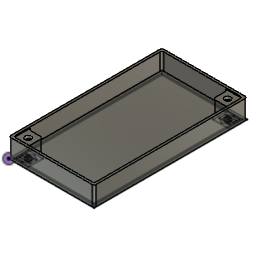
assemblage v25 (Autodesk Fusion 360 archive; units mm, degrees)
design "basBoite"
Autodesk Fusion 360 part; units mm, degrees
sketch "Sketch1" plane through (0, 0, 0) normal (0, 0, 1) x (1, 0, 0)
  line L0 (0, 0) -> (44, 0)
  line L1 (44, 0) -> (44, 79)
  line L2 (44, 79) -> (0, 79)
  line L3 (0, 79) -> (0, 0)
  line L4 (1.2, 1.2) -> (42.8, 1.2)
  line L5 (42.8, 1.2) -> (42.8, 77.8)
  line L6 (42.8, 77.8) -> (1.2, 77.8)
  line L7 (1.2, 77.8) -> (1.2, 1.2)
  line L8 (42, 2) -> (42, 77)
  line L9 (42, 77) -> (2, 77)
  line L10 (2, 77) -> (2, 2)
  line L11 (2, 2) -> (42, 2)
  line L12 (1.2, 1.2) -> (8.8, 1.2)
  line L13 (8.8, 1.2) -> (8.8, 8.8)
  line L14 (8.8, 8.8) -> (1.2, 8.8)
  line L15 (1.2, 8.8) -> (1.2, 1.2)
  line L16 (2, 2) -> (5, 2)
  line L17 (5, 2) -> (5, 5)
  line L18 (5, 5) -> (2, 5)
  line L19 (2, 5) -> (2, 2)
  circle A0 centre (5, 5) radius 1.6
  line L20 (7.75, 6.5877) -> (5, 8.1754)
  line L21 (5, 8.1754) -> (2.25, 6.5877)
  line L22 (2.25, 6.5877) -> (2.25, 3.4123)
  line L23 (2.25, 3.4123) -> (5, 1.8246)
  line L24 (5, 1.8246) -> (7.75, 3.4123)
  line L25 (7.75, 3.4123) -> (7.75, 6.5877)
  line L26 (2.25, 6.6) -> (7.75, 6.6)
  line L27 (2.25, 3.4) -> (7.75, 3.4)
  line L28 (6.6, 6.6) -> (6.6, 3.4)
  line L29 (3.4, 6.6) -> (3.4, 3.4)
  line L30 (42.8, 77.8) -> (35.2, 77.8)
  line L31 (35.2, 77.8) -> (35.2, 70.2)
  line L32 (35.2, 70.2) -> (42.8, 70.2)
  line L33 (42.8, 70.2) -> (42.8, 77.8)
  line L34 (42, 77) -> (39, 77)
  line L35 (39, 77) -> (39, 74)
  line L36 (39, 74) -> (42, 74)
  line L37 (42, 74) -> (42, 77)
  circle A1 centre (39, 74) radius 1.6
  line L38 (36.25, 72.4123) -> (39, 70.8246)
  line L39 (39, 70.8246) -> (41.75, 72.4123)
  line L40 (41.75, 72.4123) -> (41.75, 75.5877)
  line L41 (41.75, 75.5877) -> (39, 77.1754)
  line L42 (39, 77.1754) -> (36.25, 75.5877)
  line L43 (36.25, 75.5877) -> (36.25, 72.4123)
  line L44 (36.25, 75.6) -> (41.75, 75.6)
  line L45 (36.25, 72.4) -> (41.75, 72.4)
  line L46 (37.4, 75.6) -> (37.4, 72.4)
  line L47 (40.6, 75.6) -> (40.6, 72.4)
  point P0 (5, 5)
  point P1 (39, 74)
  dimension "d1" = 44
  dimension "d2" = 79
  dimension "d3" = -1.2
  dimension "d4" = -2
  dimension "d35" = 7.6
  dimension "d36" = 7.6
  dimension "d37" = 3
  dimension "d38" = 3
  dimension "d39" = 3.2
  dimension "d40" = 2.75
  dimension "d41" = 7.6
  dimension "d42" = 7.6
  dimension "d43" = 3
  dimension "d44" = 3
  dimension "d45" = 3.2
  dimension "d46" = 2.75
  constraint horizontal L0
  constraint vertical L1
  constraint horizontal L2
  constraint vertical L3
  constraint coincident L0.start L3.end
  constraint horizontal L12
  constraint vertical L13
  constraint horizontal L14
  constraint vertical L15
  constraint horizontal L16
  constraint vertical L17
  constraint horizontal L18
  constraint vertical L19
  constraint coincident P0 L17.end
  constraint coincident L22 L26.start
  constraint coincident L25 L26.end
  constraint perpendicular L25 L26
  constraint coincident L22 L27.start
  constraint coincident L25 L27.end
  constraint perpendicular L25 L27
  constraint tangent A0 L26
  constraint tangent A0 L27
  constraint coincident L26 L28.start
  constraint coincident L27 L28.end
  constraint perpendicular L27 L28
  constraint coincident L26 L29.start
  constraint coincident L27 L29.end
  constraint perpendicular L27 L29
  constraint tangent A0 L29
  constraint tangent A0 L28
  constraint horizontal L30
  constraint vertical L31
  constraint horizontal L32
  constraint vertical L33
  constraint horizontal L34
  constraint vertical L35
  constraint horizontal L36
  constraint vertical L37
  constraint coincident P1 L35.end
  constraint coincident L43 L44.start
  constraint coincident L40 L44.end
  constraint perpendicular L40 L44
  constraint coincident L43 L45.start
  constraint coincident L40 L45.end
  constraint perpendicular L40 L45
  constraint tangent A1 L44
  constraint tangent A1 L45
  constraint coincident L44 L46.start
  constraint coincident L45 L46.end
  constraint perpendicular L45 L46
  constraint coincident L44 L47.start
  constraint coincident L45 L47.end
  constraint perpendicular L45 L47
  constraint tangent A1 L46
  constraint tangent A1 L47
  constraint vertical L25
  constraint vertical L43
  measures "d1" distance of L0.start L0.end
  measures "d2" distance of L0.start L2.end
  measures "d35" distance of L4.start L12.end
  measures "d36" distance of L4.start L14.end
  measures "d37" distance of L10.end L16.end
  measures "d38" distance of L10.end L18.end
  measures "d39" diameter of A0
  measures "d40" distance of P0 L25
  measures "d41" distance of L5.end L30.end
  measures "d42" distance of L5.end L32.end
  measures "d43" distance of L8.end L34.end
  measures "d44" distance of L8.end L36.end
  measures "d45" diameter of A1
  measures "d46" distance of P1 L43
extrude "Extrude21" add sketch "Sketch1" along normal blind 1.2 contours L4 L5 L8 L11 L13 L32 | L6 L7 L9 L10 L14 L31 | L8 L9 L10 L11 L13 L14 L31 L32
extrude "Extrude22" add sketch "Sketch1" along normal blind 10
extrude "Extrude23" add sketch "Sketch1" along normal blind 9 contours L5 L6 L8 L9 L30 L31 L32 L33 L34 L37 L41 L42 | L8 L9 L31 L32 L36 L38 L39 L40 L42 L43 | L8 L9 L34 L36 L37 L40 L41 | L9 L35 L42 L44 | L36 L39 L40 L45 L47 | L36 L40 L41 L44 L47 | L9 L34 L35 L41 L44 | L38 L42 L43 L44 L45 L46 | A1 L45 L47 | A1 L44 L47 | A1 L44 L46 | A1 L45 L46 | L38 L39 L45
extrude "Extrude24" add sketch "Sketch1" along normal blind 9 contours L9 L34 L41 L42
extrude "Extrude25" cut sketch "Sketch1" along normal blind 7.8 contours A1 L45 L47 | A1 L44 L47 | A1 L44 L46 | A1 L45 L46
extrude "Extrude26" cut sketch "Sketch1" along normal blind 7.5 contours L36 L39 L40 L45 L47 | L36 L40 L41 L44 L47 | L38 L42 L43 L44 L45 L46
extrude "Extrude27" cut sketch "Sketch1" along normal blind 7.2 contours L9 L34 L41 L42 | L9 L35 L42 L44 | L9 L34 L35 L41 L44 | L38 L39 L45
extrude "Extrude28" add sketch "Sketch1" along normal blind 9 contours L4 L7 L10 L11 L12 L13 L14 L15 L16 L19 L23 L24 | L10 L11 L13 L14 L18 L20 L21 L22 L24 L25 | L11 L16 L23 L24 | L11 L17 L24 L27 | L10 L11 L16 L18 L19 L22 L23 | L11 L16 L17 L23 L27 | L20 L24 L25 L26 L27 L28 | L18 L21 L22 L26 L29 | L18 L22 L23 L27 L29 | A0 L27 L29 | A0 L27 L28 | A0 L26 L29 | A0 L26 L28 | L20 L21 L26
extrude "Extrude29" cut sketch "Sketch1" along normal blind 7.8 contours A0 L27 L29 | A0 L27 L28 | A0 L26 L29 | A0 L26 L28
extrude "Extrude30" cut sketch "Sketch1" along normal blind 7.5 contours L20 L24 L25 L26 L27 L28 | L18 L21 L22 L26 L29 | L18 L22 L23 L27 L29
extrude "Extrude31" cut sketch "Sketch1" along normal blind 7.2 contours L11 L16 L23 L24 | L11 L17 L24 L27 | L11 L16 L17 L23 L27 | L20 L21 L26
extrude "Extrude33" cut 1 faces at (0.4, 52.2667, 10) along direction (0, 0, -1) blind 0.1
fillet "Fillet6" radius 1 11 edges at (1.2, 77.8, 5.55) (35.2, 70.2, 5.1) (35.2, 77.8, 5.1) (42.8, 70.2, 5.1) (1.2, 8.8, 5.1) (8.8, 1.2, 5.1) (8.8, 8.8, 5.1) (0, 79, 4.95) (44, 0, 4.95) (44, 79, 4.95) (0, 0, 4.95)
fillet "Fillet7" radius 1 2 edges at (42.8, 1.2, 5.55) (1.2, 1.2, 9.45)
extrude "Extrude34" add 1 faces at (4.9601, 8.0652, 9) along direction (0, 0, 1) blind 0.3
extrude "Extrude35" add 1 faces at (39.0399, 70.9348, 9) along direction (0, 0, 1) blind 0.3
fillet "Fillet8" radius 1 1 edges at (42.8, 77.8, 9.6)
